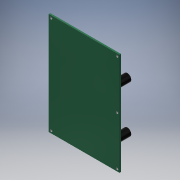
# Autodesk Inventor part: 13090모터드라이브
Saved by Autodesk Inventor 2017 (Build 210142000, 142)
## iProperties
Part Number: 13090모터드라이브
Material: 일반
Document SubType Name: Modeling
Designer: minom
Density: 1 g/cm^3
Appearance: 기본값
Author: minom
Autodesk Inventor part; units mm, degrees
ref_plane "YZ Plane" through (0, 0, 0) normal (1, 0, 0) x (0, 1, 0)
ref_plane "XZ Plane" through (0, 0, 0) normal (0, 1, 0) x (-1, 0, 0)
ref_plane "XY Plane" through (0, 0, 0) normal (0, 0, 1) x (1, 0, 0)
sketch "스케치1" plane through (0, 0, 0) normal (0, 1, 0) x (-1, 0, 0)
  line L0 (0, 0) -> (-90, 0)
  line L1 (-90, 0) -> (-90, -130)
  line L2 (-90, -130) -> (0, -130)
  line L3 (0, -130) -> (0, 0)
  dimension "d0" = 90
  dimension "d1" = 130
  constraints: 8 end point, 2 parallel, 1 horizontal, 1 perpendicular
  measures "d0" distance of L2.end L1.end
  measures "d1" distance of L1.end L0.end
extrude "돌출1" add sketch "스케치1" along normal blind 2
sketch "스케치2" plane through (0, 2, 0) normal (0, 1, 0) x (1, 0, 0)
  circle A0 centre (85, 95) radius 5
  circle A1 centre (85, 35) radius 5
  line L0 (0, 0) -> (90, 0) projected
  line L1 (90, 0) -> (90, 130) projected
  line L2 (90, 130) -> (0, 130) projected
  line L3 (0, 130) -> (0, 0) projected
  circle A2 centre (15, 105) radius 5
  circle A3 centre (15, 95) radius 5
  circle A4 centre (15, 35) radius 5
  circle A5 centre (15, 25) radius 5
  dimension "d4" = 10
  dimension "d5" = 10
  dimension "d6" = 5
  dimension "d7" = 5
  dimension "d8" = 35
  dimension "d9" = 35
  dimension "d10" = 10
  dimension "d11" = 10
  dimension "d12" = 10
  dimension "d13" = 10
  dimension "d14" = 25
  dimension "d15" = 10
  dimension "d16" = 25
  dimension "d17" = 10
  dimension "d18" = 15
  dimension "d19" = 15
  dimension "d20" = 15
  dimension "d21" = 15
  constraints: 6 centre point
  measures "d4" diameter of A0
  measures "d5" diameter of A1
  measures "d6" distance from line of L1 A0.centre
  measures "d7" distance from line of L1 A1.centre
  measures "d8" distance from line of A0.centre L2
  measures "d9" distance from line of L0 A1.centre
  measures "d10" diameter of A2
  measures "d11" diameter of A3
  measures "d12" diameter of A4
  measures "d13" diameter of A5
  measures "d14" distance from line of L2 A2.centre
  measures "d15" distance of A3.centre A2.centre
  measures "d16" distance from line of L0 A5.centre
  measures "d17" distance of A5.centre A4.centre
  measures "d18" distance from line of L3 A2.centre
  measures "d19" distance from line of L3 A3.centre
  measures "d20" distance from line of L3 A4.centre
  measures "d21" distance from line of L3 A5.centre
extrude "돌출2" add sketch "스케치2" along normal blind 13 contours A0 | A1 | A2 | A3 | A4 | A5
sketch "스케치3" plane through (0, 2, 0) normal (0, 1, 0) x (1, 0, 0)
  circle A0 centre (87, 127) radius 1.5
  circle A1 centre (87, 65) radius 1.5
  circle A2 centre (87, 3) radius 1.5
  line L0 (90, 0) -> (90, 130) projected
  line L1 (90, 130) -> (0, 130) projected
  line L2 (0, 0) -> (90, 0) projected
  circle A3 centre (3, 127) radius 1.5
  circle A4 centre (3, 3) radius 1.5
  line L3 (0, 130) -> (0, 0) projected
  dimension "d24" = 3
  dimension "d25" = 3
  dimension "d26" = 3
  dimension "d27" = 3
  dimension "d28" = 3
  dimension "d29" = 3
  dimension "d30" = 3
  dimension "d31" = 3
  dimension "d32" = 62
  dimension "d33" = 3
  dimension "d34" = 3
  dimension "d35" = 3
  dimension "d36" = 3
  dimension "d37" = 3
  dimension "d38" = 3
  constraints: 5 centre point
  measures "d24" diameter of A0
  measures "d25" diameter of A1
  measures "d26" diameter of A2
  measures "d27" distance from line of L0 A0.centre
  measures "d28" distance from line of L1 A0.centre
  measures "d29" distance from line of L2 A2.centre
  measures "d30" distance from line of L0 A2.centre
  measures "d31" distance from line of L0 A1.centre
  measures "d32" distance of A0.centre A1.centre
  measures "d33" diameter of A3
  measures "d34" diameter of A4
  measures "d35" distance from line of L3 A3.centre
  measures "d36" distance from line of L1 A3.centre
  measures "d37" distance from line of L2 A4.centre
  measures "d38" distance from line of L3 A4.centre
extrude "돌출3" cut sketch "스케치3" against normal blind 2 contours A0 | A1 | A2 | A3 | A4
